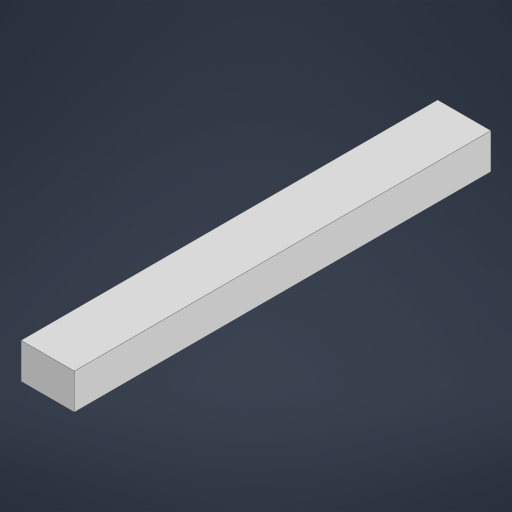
# Autodesk Inventor part: MotorNatazkaPodkladka
Saved by Autodesk Inventor 2024 (Build 280153000, 153)
## iProperties
Created: 2023-11-07
Part Number: MotorNatazkaPodkladka
Material: Generic
Document SubType Name: Modeling
Designer: KirikDK
Density: 1 g/cm^3
Appearance: Default
Mass: 140.7 g
Surface Area: 246.5 cm^2
Volume: 140.7 cm^3
Author: KirikDK
Autodesk Inventor part; units mm, degrees
ref_plane "YZ Plane" through (0, 0, 0) normal (1, 0, 0) x (0, 1, 0)
ref_plane "XZ Plane" through (0, 0, 0) normal (0, 1, 0) x (-1, 0, 0)
ref_plane "XY Plane" through (0, 0, 0) normal (0, 0, 1) x (1, 0, 0)
sketch "Sketch1" plane through (0, 0, 0) normal (0, 1, 0) x (-1, 0, 0)
  line L0 (22.5, 45) -> (-7.5, 45)
  line L1 (-7.5, 45) -> (-7.5, -189.5)
  line L2 (-7.5, -189.5) -> (22.5, -189.5)
  line L3 (22.5, -189.5) -> (22.5, 45)
  point P0 (0, 0)
  dimension "d0" = 30
  dimension "d1" = 234.5
  constraints: 8 end point, 2 parallel, 1 horizontal, 1 perpendicular
  measures "d0" distance of L0.start L0.end
  measures "d1" distance of L2.end L0.start
extrude "Extrusion1" add sketch "Sketch1" along normal blind 20
body "Solid1"
